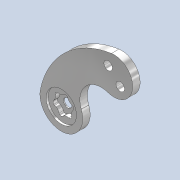
# Autodesk Inventor part: 原動節2
Saved by Autodesk Inventor 2020.4 (Build 244396000, 396)
## iProperties
Created: 2021-04-23
Part Number: 原動節2
Material: アルミニウム 2014-T4
Document SubType Name: Modeling
Designer: happy
Density: 2.8 g/cm^3
Appearance: サテン
Mass: 7.56237 g
Surface Area: 23.7289 cm^2
Volume: 2.70085 cm^3
Author: happy
Autodesk Inventor part; units mm, degrees
ref_plane "YZ Plane" through (0, 0, 0) normal (1, 0, 0) x (0, 1, 0)
ref_plane "XZ Plane" through (0, 0, 0) normal (0, 1, 0) x (-1, 0, 0)
ref_plane "XY Plane" through (0, 0, 0) normal (0, 0, 1) x (1, 0, 0)
sketch "スケッチ1" plane through (0, 0, 0) normal (0, 0, 1) x (1, 0, 0)
  line L0 (0, 0) -> (24.7487, 24.7487) construction
  line L1 (0, 0) -> (8.6903, 0) construction
  circle A0 centre (7.0711, 7.0711) radius 1.75 construction
  circle A1 centre (12.0208, 12.0208) radius 1.75 construction
  circle A2 centre (24.7487, 24.7487) radius 4.6188 construction
  circle A3 centre (24.7487, 24.7487) radius 8.6188
  line L2 (21.4828, 21.4828) -> (28.0147, 28.0147) construction
  circle A4 centre (29.2102, 23.5533) radius 4 construction
  circle A5 centre (21.4828, 21.4828) radius 4 construction
  circle A6 centre (23.5533, 29.2102) radius 4 construction
  circle A7 centre (29.2102, 23.5533) radius 1.25
  circle A8 centre (21.4828, 21.4828) radius 1.25
  circle A9 centre (23.5533, 29.2102) radius 1.25
  circle A10 centre (24.7487, 24.7487) radius 0.8755 construction
  circle A11 centre (0, 0) radius 5 construction
  arc A12 (5.7301, 8.1955) -> (7.0711, 7.0711) centre (0, 0) ccw
  arc A13 (21.9392, 16.6007) -> (9.3397, 3.5735) centre (18.6794, 7.1469) ccw
  line L3 (-4.8296, -1.2941) -> (-3.5355, 3.5355) construction
  line L4 (-3.5355, 3.5355) -> (1.2941, 4.8296) construction
  line L5 (1.2941, 4.8296) -> (4.8296, 1.2941) construction
  line L6 (4.8296, 1.2941) -> (3.5355, -3.5355) construction
  line L7 (3.5355, -3.5355) -> (-1.2941, -4.8296) construction
  line L8 (-1.2941, -4.8296) -> (-4.8296, -1.2941) construction
  arc A14 (-2.5213, 3.8073) -> (-3.8073, 2.5213) centre (-2.7931, 2.7931) ccw
  arc A15 (-4.5579, -0.2799) -> (-4.0872, -2.0366) centre (-3.8154, -1.0223) ccw
  arc A16 (-2.0366, -4.0872) -> (-0.2799, -4.5579) centre (-1.0223, -3.8154) ccw
  arc A17 (2.5213, -3.8073) -> (3.8073, -2.5213) centre (2.7931, -2.7931) ccw
  arc A18 (4.5579, 0.2799) -> (4.0872, 2.0366) centre (3.8154, 1.0223) ccw
  arc A19 (2.0366, 4.0872) -> (0.2799, 4.5579) centre (1.0223, 3.8154) ccw
  arc A20 (-2.5213, 3.8073) -> (0.2799, 4.5579) centre (-1.7707, 6.6085) ccw
  arc A21 (-4.5579, -0.2799) -> (-3.8073, 2.5213) centre (-6.6085, 1.7707) ccw
  arc A22 (-2.0366, -4.0872) -> (-4.0872, -2.0366) centre (-4.8377, -4.8377) ccw
  arc A23 (2.5213, -3.8073) -> (-0.2799, -4.5579) centre (1.7707, -6.6085) ccw
  arc A24 (4.5579, 0.2799) -> (3.8073, -2.5213) centre (6.6085, -1.7707) ccw
  arc A25 (2.0366, 4.0872) -> (4.0872, 2.0366) centre (4.8377, 4.8377) ccw
  circle A26 centre (0, 0) radius 7.1
  arc A27 (23.49, 33.2751) -> (-9.7773, 2.0987) centre (29.3319, -6.296) ccw
  line L9 (24.7487, 24.7487) -> (104.2613, 104.2613)
  circle A28 centre (24.7487, 24.7487) radius 4 construction
  circle A29 centre (24.7487, 24.7487) radius 8
  line L10 (26.6251, 21.2161) -> (22.8724, 28.2813) construction
  circle A30 centre (27.5772, 21.9203) radius 4 construction
  circle A31 centre (21.9203, 27.5772) radius 4 construction
  circle A32 centre (27.5772, 21.9203) radius 3
  circle A33 centre (21.9203, 27.5772) radius 3
  line L11 (27.5772, 21.9203) -> (21.9203, 27.5772) construction
  circle A34 centre (27.5772, 21.9203) radius 2
  circle A35 centre (21.9203, 27.5772) radius 2
  point P0 (220.0202, -53)
  point P1 (1.1978, 9.928)
  point P2 (16.1509, 24.1477)
  point P3 (-4.8296, -1.2941)
  point P4 (-1.2941, -4.8296)
  point P5 (3.5355, -3.5355)
  point P6 (4.8296, 1.2941)
  point P7 (4.0872, 2.0366)
  point P8 (4.5579, 0.2799)
  point P9 (3.8073, -2.5213)
  point P10 (2.5213, -3.8073)
  point P11 (-0.2799, -4.5579)
  point P12 (-2.0366, -4.0872)
  point P13 (-4.0872, -2.0366)
  point P14 (-4.5579, -0.2799)
  point P15 (9.6734, 11.4934)
  point P16 (9.9876, 0.4979)
  dimension "d2" = 3.5
  dimension "d15" = 10
  dimension "d0" = 35
  dimension "d1" = 45
  dimension "d3" = 3.5
  dimension "d4" = 10
  dimension "d5" = 7
  dimension "d10" = 17.2376
  dimension "d11" = 8
  dimension "d13" = 2.5
  dimension "d16" = 20
  dimension "d22" = 360
  dimension "d26" = 360
  dimension "d28" = 1.05
  dimension "d29" = 14.2
  dimension "d35" = 11
  dimension "d37" = 40
  dimension "d38" = 10
  dimension "d43" = 16
  dimension "d44" = 8
  dimension "d45" = 6
  dimension "d46" = 6
  dimension "d47" = 4
  dimension "d48" = 4
  constraints: 54 point on circle, 34 centre point, 24 end point, 16 coincident, 13 tangent, 6 point on line, 5 equal radius, 5 midpoint, 1 collinear, 1 concentric, 1 horizontal, 1 perpendicular, 75 other
  measures "d0" distance of L0.start L0.end
  measures "d1" angle of L1 L0
  measures "d3" diameter of A1
  measures "d4" distance of L0.start point (7.071, 7.071)
  measures "d5" distance of A1.centre point (7.071, 7.071)
  measures "d10" diameter of A3
  measures "d11" diameter of A5
  measures "d13" diameter of A8
  measures "d16" diameter of A12
  measures "d28" radius of A14
  measures "d29" diameter of A26
  measures "d35" distance of point (9.988, 0.498) point (9.673, 11.493)
  measures "d37" radius of A27
  measures "d38" radius of A13
  measures "d43" diameter of A29
  measures "d44" diameter of A30
  measures "d45" diameter of A32
  measures "d46" diameter of A33
  measures "d47" diameter of A34
  measures "d48" diameter of A35
extrude "押し出し1" add sketch "スケッチ1" along normal blind 3 contours A3 | A3 A13 A12 A27 | A7 A32 | A32 A7 A34 | A7 A34 A32 | A8 | A9 A33 | A33 A9 A35 | A9 A35 A33 | A26 | A29
sketch "スケッチ2" plane through (0, 0, 3) normal (0, 0, 1) x (1, 0, 0)
  circle A0 centre (0, 0) radius 7.1 projected
extrude "押し出し2" cut sketch "スケッチ2" against normal blind 1
sketch "スケッチ3" plane through (0, 0, 0) normal (0, 0, -1) x (-1, 0, 0)
  arc A0 (-23.49, 33.2751) -> (-21.9392, 16.6007) centre (-24.7487, 24.7487) ccw projected
  arc A1 (-9.3397, 3.5735) -> (-21.9392, 16.6007) centre (-18.6794, 7.1469) ccw projected
  arc A2 (-9.3397, 3.5735) -> (9.7773, 2.0987) centre (0, 0) ccw projected
  arc A3 (9.7773, 2.0987) -> (-23.49, 33.2751) centre (-29.3319, -6.296) ccw projected
  circle A4 centre (0, 0) radius 2
  circle A5 centre (-27.5772, 21.9203) radius 2 projected
  circle A6 centre (-21.9203, 27.5772) radius 2 projected
  dimension "d39" = 4
  constraints: 1 centre point, 1 coincident
  measures "d39" diameter of A4
extrude "押し出し3" add sketch "スケッチ3" along normal blind 0.5
